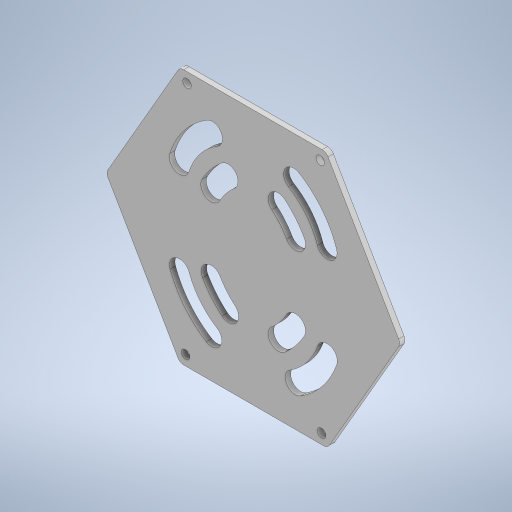
# Autodesk Inventor part: ArmPowerBoardLargerLid
Saved by Autodesk Inventor 2023 (Build 270158000, 158)
## iProperties
Created: 2023-12-03
Part Number: ArmPowerBoardLargerLid
Material: Generic
Document SubType Name: Sheet Metal
Designer: LattePanda
Density: 1 g/cm^3
Sheet Metal Rule: Default
Appearance: Default
Author: LattePanda
Autodesk Inventor part; units mm, degrees
ref_plane "YZ Plane" through (0, 0, 0) normal (1, 0, 0) x (0, 1, 0)
ref_plane "XZ Plane" through (0, 0, 0) normal (0, 1, 0) x (-1, 0, 0)
ref_plane "XY Plane" through (0, 0, 0) normal (0, 0, 1) x (1, 0, 0)
sketch "Sketch1" plane through (0, 0, 0) normal (0, 0, 1) x (1, 0, 0)
  line L0 (-0.5774, 75.2102) -> (-21.4226, 39.1051)
  circle A0 centre (2.1485, 73.2102) radius 1.25
  arc A1 (1.1547, 76.2102) -> (-0.5774, 75.2102) centre (1.1547, 74.2102) ccw
  line L1 (42.4288, 76.2102) -> (1.1547, 76.2102)
  arc A2 (44.1609, 75.2102) -> (42.4288, 76.2102) centre (42.4288, 74.2102) ccw
  line L2 (65.2144, 38.7444) -> (44.1609, 75.2102)
  circle A3 centre (41.8515, 73.2102) radius 1.25
  arc A4 (65.2144, 36.7444) -> (65.2144, 38.7444) centre (63.4824, 37.7444) ccw
  line L3 (44.5774, 1) -> (65.2144, 36.7444)
  arc A5 (42.8453, 0) -> (44.5774, 1) centre (42.8453, 2) ccw
  line L4 (1.1547, 0) -> (42.8453, 0)
  arc A6 (-0.5774, 1) -> (1.1547, 0) centre (1.1547, 2) ccw
  line L5 (-21.4226, 37.1051) -> (-0.5774, 1)
  circle A7 centre (1.7321, 3) radius 1.25
  circle A8 centre (42.2679, 3) radius 1.25
  arc A9 (-21.4226, 39.1051) -> (-21.4226, 37.1051) centre (-19.6906, 38.1051) ccw
  point P0 (0, 0)
  point P1 (22, 38.1051)
  dimension "d0" = 2
  dimension "d1" = 2.5
  dimension "d2" = 120
  dimension "d3" = 120
  dimension "d4" = 75.8495
  dimension "d5" = 76.2102
  dimension "d6" = 76.2102
  dimension "d7" = 75.8495
  dimension "d8" = 38.1051
  dimension "d9" = 76.2102
  dimension "d10" = 37.7444
  dimension "d11" = 3
  dimension "d12" = 3
  dimension "d13" = 38.4658
  dimension "d14" = 37.7444
  dimension "d15" = 38.1051
  dimension "d16" = 37.3837
  dimension "d17" = 72.8495
  dimension "d18" = 72.8495
  dimension "d19" = 38.1051
  measures "d0" radius of A4
  measures "d1" diameter of A8
  measures "d2" angle of L2 L3
  measures "d3" angle of L2 L1
  measures "d4" distance between parallel lines of L2 L5
  measures "d5" distance between parallel lines of L3 L0
  measures "d6" distance between parallel lines of L1 L4
  measures "d7" distance from line of point (0, 0) L2
  measures "d8" distance from line of point (0, 0) L3
  measures "d9" distance from line of point (0, 0) L1
  measures "d10" distance from line of A8.centre L2
  measures "d11" distance from line of A8.centre L3
  measures "d12" distance from line of A3.centre L2
  measures "d13" distance from line of A3.centre L3
  measures "d14" distance from line of point (22, 38.105) L2
  measures "d15" distance from line of point (22, 38.105) L3
  measures "d16" distance from line of A0.centre L2
  measures "d17" distance from line of A0.centre L3
  measures "d18" distance from line of A7.centre L2
  measures "d19" distance from line of A7.centre L3
extrude "Plate1" add sketch "Sketch1" along normal blind 1.6002
sketch "Sketch2" plane through (0, 0, 1.6002) normal (0, 0, 1) x (1, 0, 0)
  arc A0 (43.8587, 51.7336) -> (33.9602, 64.2102) centre (21.8785, 44.4602) ccw construction
  arc A1 (46.7068, 52.676) -> (35.5257, 66.7694) centre (21.8785, 44.4602) ccw
  arc A2 (41.0106, 50.7911) -> (32.3947, 61.6511) centre (21.8785, 44.4602) ccw
  arc A3 (41.0106, 50.7911) -> (46.7068, 52.676) centre (43.8587, 51.7336) ccw
  arc A4 (35.5257, 66.7694) -> (32.3947, 61.6511) centre (33.9602, 64.2102) ccw
  arc A5 (34.4317, 12) -> (43.9348, 23.8871) centre (21.9132, 31.75) ccw construction
  arc A6 (36.0378, 9.4661) -> (46.7601, 22.8783) centre (21.9132, 31.75) ccw
  arc A7 (32.8256, 14.5339) -> (41.1095, 24.8959) centre (21.9132, 31.75) ccw
  arc A8 (32.8256, 14.5339) -> (36.0378, 9.4661) centre (34.4317, 12) ccw
  arc A9 (46.7601, 22.8783) -> (41.1095, 24.8959) centre (43.9348, 23.8871) ccw
  line L0 (42.4288, 76.2102) -> (1.1547, 76.2102) construction
  line L1 (21.7918, 76.2102) -> (22, 0) construction
  line L2 (1.1547, 0) -> (42.8453, 0) construction
  line L3 (44.1609, 75.2102) -> (65.2144, 38.7444) construction
  line L4 (65.2144, 36.7444) -> (44.5774, 1) construction
  line L5 (43.9348, 23.8871) -> (43.8587, 51.7336) construction
  arc A10 (8.1096, 66.6945) -> (-2.9943, 52.5402) centre (21.8785, 44.4602) ccw
  arc A11 (11.2685, 61.5934) -> (2.7121, 50.6864) centre (21.8785, 44.4602) ccw
  arc A12 (-2.9943, 52.5402) -> (2.7121, 50.6864) centre (-0.1411, 51.6133) ccw
  arc A13 (11.2685, 61.5934) -> (8.1096, 66.6945) centre (9.689, 64.1439) ccw
  arc A14 (-2.8848, 22.7426) -> (7.9107, 9.3893) centre (21.9132, 31.75) ccw
  arc A15 (2.7547, 24.7911) -> (11.0951, 14.4745) centre (21.9132, 31.75) ccw
  arc A16 (7.9107, 9.3893) -> (11.0951, 14.4745) centre (9.5029, 11.9319) ccw
  arc A17 (2.7547, 24.7911) -> (-2.8848, 22.7426) centre (-0.065, 23.7669) ccw
  arc A18 (34.4623, 49.3127) -> (29.3604, 55.511) centre (14.3066, 37.9208) ccw construction
  arc A19 (37.0741, 50.7888) -> (31.311, 57.7902) centre (14.3066, 37.9208) ccw
  arc A20 (31.8506, 47.8365) -> (27.4097, 53.2317) centre (14.3066, 37.9208) ccw
  arc A21 (31.8506, 47.8365) -> (37.0741, 50.7888) centre (34.4623, 49.3127) ccw
  arc A22 (31.311, 57.7902) -> (27.4097, 53.2317) centre (29.3604, 55.511) ccw
  line L6 (21.8785, 44.4602) -> (40.0161, 58.8498) construction
  arc A23 (-21.4226, 39.1051) -> (-21.4226, 37.1051) centre (-19.6906, 38.1051) ccw projected
  line L7 (21.8959, 38.1051) -> (61.5151, 38.1051) construction
  arc A24 (65.2144, 36.7444) -> (65.2144, 38.7444) centre (63.4824, 37.7444) ccw projected
  arc A25 (31.311, 18.42) -> (37.0741, 25.4214) centre (14.3066, 38.2894) ccw
  arc A26 (27.4097, 22.9786) -> (31.8506, 28.3737) centre (14.3066, 38.2894) ccw
  arc A27 (37.0741, 25.4214) -> (31.8506, 28.3737) centre (34.4623, 26.8976) ccw
  arc A28 (27.4097, 22.9786) -> (31.311, 18.42) centre (29.3604, 20.6993) ccw
  arc A29 (12.3733, 57.7385) -> (6.6486, 50.7057) centre (29.4861, 37.9623) ccw
  arc A30 (16.2994, 53.2013) -> (11.8881, 47.782) centre (29.4861, 37.9623) ccw
  arc A31 (6.6486, 50.7057) -> (11.8881, 47.782) centre (9.2683, 49.2438) ccw
  arc A32 (16.2994, 53.2013) -> (12.3733, 57.7385) centre (14.3364, 55.4699) ccw
  arc A33 (12.5885, 18.3688) -> (16.4648, 22.9486) centre (14.5266, 20.6587) ccw
  arc A34 (6.7872, 25.3387) -> (12.5885, 18.3688) centre (29.4841, 38.3309) ccw
  arc A35 (11.9945, 28.3194) -> (16.4648, 22.9486) centre (29.4841, 38.3309) ccw
  arc A36 (11.9945, 28.3194) -> (6.7872, 25.3387) centre (9.3908, 26.8291) ccw
  point P0 (0, 0)
  point P1 (32.1821, 52.6346)
  dimension "d21" = 12
  dimension "d22" = 12
  dimension "d23" = 3
  dimension "d24" = 12
  dimension "d25" = 12
  dimension "d26" = 31.75
  dimension "d27" = 31.75
  dimension "d28" = 22
  dimension "d29" = 10
  dimension "d30" = 31.3924
  dimension "d31" = 18.3481
  constraints: 73 point on circle, 35 centre point, 33 symmetric about line, 12 tangent, 8 end point, 3 equal radius, 3 midpoint, 3 point on line, 1 horizontal, 1 parallel, 20 other
  measures "d21" distance from line of L0 A0.end
  measures "d22" distance from line of L2 A5.start
  measures "d23" radius of A4
  measures "d24" distance from line of L3 L5.end
  measures "d25" distance from line of L4 L5.start
  measures "d26" distance from line of L0 L6.start
  measures "d27" distance from line of L2 A5.centre
  measures "d28" distance between parallel lines of L1 L5
  measures "d29" distance of point (32.182, 52.635) L6.end
  measures "d30" distance from line of A19.start L4
  measures "d31" distance from line of A19.start L3
extrude "Cut1" cut sketch "Sketch2" against normal blind 1.6002
equation "\"d22\" = d21"
equation "\"d24\" = d21"
equation "\"d25\" = d21"
equation "\"d27\" = d26"
equation "\"d32\" = Thickness"
equation "\"d20\" = Thickness"
equation "\"BendRadius\" = Thickness"
equation "\"BendReliefWidth\" = Thickness"
equation "\"BendReliefDepth\" = 0.5 * Thickness"
equation "\"CornerReliefSize\" = 4 * Thickness"
equation "\"MinimumRemnant\" = 2 * Thickness"
equation "\"TransitionRadius\" = BendRadius"
equation "\"JacobiRadiusSize\" = BendRadius"
equation "\"GapSize\" = Thickness"
equation "\"Thickness\" = 1.6002"
body "Solid1"
